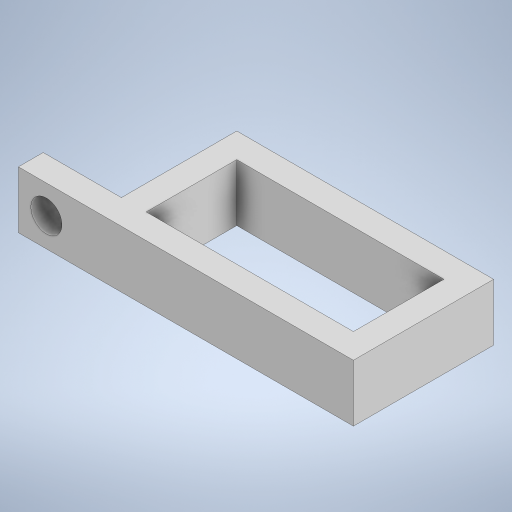
# Autodesk Inventor part: Switch_Holder
Saved by Autodesk Inventor 2023 (Build 270158000, 158)
## iProperties
Created: 2022-09-28
Part Number: Switch_Holder
Material: Generic
Document SubType Name: Sheet Metal
Designer: Windows10
Density: 1 g/cm^3
Sheet Metal Rule: Default_mm
Appearance: Default
Author: Windows10
Autodesk Inventor part; units mm, degrees
ref_plane "YZ Plane" through (0, 0, 0) normal (1, 0, 0) x (0, 1, 0)
ref_plane "XZ Plane" through (0, 0, 0) normal (0, 1, 0) x (-1, 0, 0)
ref_plane "XY Plane" through (0, 0, 0) normal (0, 0, 1) x (1, 0, 0)
sketch "Sketch1" plane through (0, 0, 0) normal (0, 0, 1) x (1, 0, 0)
  line L0 (0, 0) -> (27, 0)
  line L1 (27, 0) -> (27, -4.6)
  line L2 (27, -4.6) -> (0, -4.6)
  line L3 (0, -4.6) -> (0, 0)
  circle A0 centre (2.2589, -2.3) radius 1.25
  dimension "d0" = 2.3
  dimension "d1" = 2.3
  dimension "d2" = 27
  dimension "d12" = 2.5
  constraints: 8 end point, 2 parallel, 1 centre point, 1 horizontal, 1 perpendicular
  measures "d0" distance from line of L0 A0.centre
  measures "d1" distance from line of L2 A0.centre
  measures "d2" distance of L1.end L2.end
  measures "d12" diameter of A0
extrude "Extrusion1" add sketch "Sketch1" along normal blind 2
sketch "Sketch2" plane through (0, 0, 0) normal (0, 0, -1) x (-1, 0, 0)
  line L0 (0, -4.6) -> (-27, -4.6) projected
  line L1 (-6.3, 0) -> (-8.3, 0)
  line L2 (-8.3, 0) -> (-8.3, -4.6)
  line L3 (-8.3, -4.6) -> (-6.3, -4.6)
  line L4 (-6.3, -4.6) -> (-6.3, 0)
  line L5 (-27, 0) -> (0, 0) projected
  line L6 (-27, -4.6) -> (-25, -4.6)
  line L7 (-25, -4.6) -> (-25, 0)
  line L8 (-25, 0) -> (-27, 0)
  line L9 (-27, 0) -> (-27, -4.6)
  dimension "d5" = 2
  dimension "d6" = 2
  dimension "d7" = 16.7
  constraints: 16 end point, 4 parallel, 2 horizontal, 2 perpendicular, 2 point on line
  measures "d5" distance between parallel lines of L9 L7
  measures "d6" distance between parallel lines of L2 L4
  measures "d7" distance between parallel lines of L7 L2
extrude "Extrusion2" add sketch "Sketch2" along normal blind 7.3 contours L0 L2 L1 L4 | L0 L9 L5 L7
sketch "Sketch3" plane through (0, 0, -7.3) normal (0, 0, -1) x (-1, 0, 0)
  line L0 (-6.3, 0) -> (-8.3, 0) projected
  line L1 (-8.3, 0) -> (-8.3, -4.6) projected
  line L2 (-8.3, -4.6) -> (-6.3, -4.6) projected
  line L3 (-6.3, -4.6) -> (-6.3, 0) projected
  line L4 (-27, -4.6) -> (-25, -4.6) projected
  line L5 (-25, -4.6) -> (-25, 0) projected
  line L6 (-25, 0) -> (-27, 0) projected
  line L7 (-27, 0) -> (-27, -4.6) projected
  line L8 (-8.3, 0) -> (-25, 0)
  line L9 (-25, 0) -> (-25, -4.6)
  line L10 (-25, -4.6) -> (-8.3, -4.6)
  line L11 (-8.3, -4.6) -> (-8.3, 0)
  point P0 (0, 0)
  constraints: 8 end point, 2 parallel, 1 horizontal, 1 perpendicular
extrude "Extrusion3" add sketch "Sketch3" along normal blind 2
equation "\"BendRadius\" = Thickness"
equation "\"BendReliefWidth\" = Thickness"
equation "\"BendReliefDepth\" = 0.5 * Thickness"
equation "\"CornerReliefSize\" = 4 * Thickness"
equation "\"MinimumRemnant\" = 2 * Thickness"
equation "\"TransitionRadius\" = BendRadius"
equation "\"JacobiRadiusSize\" = BendRadius"
equation "\"GapSize\" = Thickness"
equation "\"Thickness\" = 0.5"
body "Solid1"
